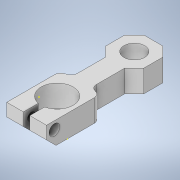
# Autodesk Inventor part: dovetail stabilizer
Saved by Autodesk Inventor 2021 (Build 250183000, 183)
## iProperties
Created: 2020-10-02
Part Number: dovetail stabilizer
Material: Generic
Document SubType Name: Modeling
Designer: User
Density: 1 g/cm^3
Appearance: Default
Author: User
Autodesk Inventor part; units mm, degrees
ref_plane "YZ Plane" through (0, 0, 0) normal (1, 0, 0) x (0, 1, 0)
ref_plane "XZ Plane" through (0, 0, 0) normal (0, 1, 0) x (-1, 0, 0)
ref_plane "XY Plane" through (0, 0, 0) normal (0, 0, 1) x (1, 0, 0)
sketch "Sketch1" plane through (0, 0, 0) normal (0, 1, 0) x (-1, 0, 0)
  line L0 (3.6632, 6.4956) -> (-8.8368, 6.4956)
  line L1 (-8.8368, 6.4956) -> (-8.8368, -10.5044)
  line L2 (-8.8368, -10.5044) -> (3.6632, -10.5044)
  line L3 (3.6632, -10.5044) -> (3.6632, 6.4956)
  line L4 (0.9132, -10.5044) -> (-6.0868, -10.5044)
  point P0 (0, 0)
  dimension "d0" = 17
  dimension "d1" = 12.5
  constraints: 10 end point, 2 horizontal, 2 parallel, 1 perpendicular, 1 point on line
  measures "d0" distance of L2.end L0.start
  measures "d1" distance of L0.start L0.end
extrude "Extrusion1" add sketch "Sketch1" along normal blind 7
chamfer "Chamfer1" distance 3 angle 45 1 edges at (2.5868, 0, 6.4956)
sketch "Sketch2" plane through (0, 7, 0) normal (0, 1, 0) x (1, 0, 0)
  circle A0 centre (2.5868, 3.1044) radius 5.025
  line L0 (8.8368, -6.4956) -> (8.8368, 10.5044) projected
  line L1 (-3.6632, -6.4956) -> (8.8368, -6.4956) projected
  point P0 (0, 0)
  dimension "d7" = 10.05
  dimension "d8" = 6.25
  dimension "d9" = 9.6
  constraints: 1 centre point
  measures "d7" diameter of A0
  measures "d8" distance from line of L0 A0.centre
  measures "d9" distance from line of L1 A0.centre
extrude "Extrusion2" cut sketch "Sketch2" against normal up to next
sketch "Sketch3" plane through (0, 7, 0) normal (0, 1, 0) x (1, 0, 0)
  line L0 (-3.6632, -6.4956) -> (8.8368, -6.4956) projected
  line L1 (1.5868, -6.4956) -> (3.5868, -6.4956)
  line L2 (3.5868, -6.4956) -> (3.5868, 0)
  line L3 (3.5868, 0) -> (1.5868, 0)
  line L4 (1.5868, 0) -> (1.5868, -6.4956)
  line L5 (8.8368, -6.4956) -> (8.8368, 10.5044) projected
  line L6 (-3.6632, 10.5044) -> (-3.6632, -6.4956) projected
  point P0 (0, 0)
  dimension "d16" = 2
  dimension "d17" = 12.5
  dimension "d18" = 5.25
  constraints: 8 end point, 2 parallel, 1 horizontal, 1 perpendicular, 1 point on line
  measures "d16" distance between parallel lines of L2 L4
  measures "d17" distance of L0.start L0.end
  measures "d18" distance between parallel lines of L5 L2
extrude "Extrusion3" cut sketch "Sketch3" against normal through all
sketch "Sketch4" plane through (8.8368, 0, -10.5044) normal (1, 0, 0) x (0, 0, -1)
  line L0 (-17, 3) -> (-17, 7) projected
  line L1 (-17, 7) -> (0, 7) projected
  point P0 (-10.5044, 0)
  point P1 (-14.5, 4.5)
  dimension "d26" = 2.5
  dimension "d27" = 2.5
  measures "d26" distance from line of L0 point (-14.5, 4.5)
  measures "d27" distance from line of L1 point (-14.5, 4.5)
hole "Hole1" at (8.8368, 4.5, 3.9956) direction (-1, 0, 0) diameter 3.4 depth 5.25 clearance for "Flat Head Machine Screw" size "M3" standard "Ansi Metric M Profile"
sketch "Sketch5" plane through (1.5868, 7, 6.4956) normal (1, 0, 0) x (0, 0, -1)
  line L0 (0, 0) -> (17, 0) projected
  line L1 (0, -4) -> (0, 0) projected
  point P0 (6.4956, -7)
  point P1 (2.5, -2.5)
  dimension "d35" = 2.5
  dimension "d36" = 2.5
  measures "d35" distance from line of L0 point (2.5, -2.5)
  measures "d36" distance from line of L1 point (2.5, -2.5)
hole "Hole2" at (1.5868, 4.5, 3.9956) direction (-1, 0, 0) diameter 2.459 depth 5.25 thread size "M3x0.5" class "6H" standard "ANSI Metric M Profile"
sketch "Sketch6" plane through (8.8368, 0, -10.5044) normal (0, 0, -1) x (-1, 0, 0)
  line L0 (5.25, 7) -> (0, 7) projected
  line L1 (3.25, 7) -> (9.25, 7)
  line L2 (9.25, 7) -> (9.25, 0)
  line L3 (9.25, 0) -> (3.25, 0)
  line L4 (3.25, 0) -> (3.25, 7)
  line L5 (0, 0) -> (0, 7) projected
  point P0 (8.8368, 0)
  dimension "d40" = 6
  dimension "d41" = 7
  dimension "d42" = 3.25
  constraints: 8 end point, 2 parallel, 1 horizontal, 1 perpendicular, 1 point on line
  measures "d40" distance of L1.start L1.end
  measures "d41" distance of L3.end L1.start
  measures "d42" distance between parallel lines of L5 L4
extrude "Extrusion4" add sketch "Sketch6" along normal blind 10.85
fillet "Fillet1" radius 2 1 edges at (8.8368, 3.5, -10.5044)
fillet "Fillet2" radius 2 1 edges at (5.5868, 3.5, -10.5044)
fillet "Fillet3" radius 2 2 edges at (-3.6632, 3.5, -10.5044) (-0.4132, 3.5, -10.5044)
sketch "Sketch7" plane through (0, 7, 0) normal (0, 1, 0) x (1, 0, 0)
  point P0 (0, 0)
sketch "Sketch8" plane through (8.8368, 0, -21.3544) normal (0, 0, -1) x (-1, 0, 0)
  point P0 (8.8368, 0)
sketch "Sketch9" plane through (0, 7, 0) normal (0, 1, 0) x (1, 0, 0)
  line L0 (5.5868, 21.3544) -> (-0.4132, 21.3544) projected
  line L1 (5.5868, 21.3544) -> (8.5868, 24.3544)
  line L2 (8.5868, 24.3544) -> (8.5868, 30.3544)
  line L3 (-3.4132, 30.3544) -> (-3.4132, 24.3544)
  line L4 (-3.4132, 24.3544) -> (-0.4132, 21.3544)
  line L5 (8.5868, 30.3544) -> (5.5868, 33.3544)
  line L6 (5.5868, 33.3544) -> (-0.4132, 33.3544)
  line L7 (-0.4132, 33.3544) -> (-3.4132, 30.3544)
  line L8 (5.5868, 12.4335) -> (5.5868, 21.3544) projected
  line L9 (-0.4132, 12.4335) -> (-0.4132, 21.3544) projected
  point P0 (0, 0)
  dimension "d110" = 6
  dimension "d111" = 6
  dimension "d112" = 6
  dimension "d113" = 6
  dimension "d114" = 45
  dimension "d115" = 135
  dimension "d116" = 45
  dimension "d117" = 45
  dimension "d118" = 45
  dimension "d119" = 3
  dimension "d120" = 3
  constraints: 14 end point, 1 horizontal, 1 perpendicular
  measures "d110" distance of L0.start L0.end
  measures "d111" distance of L5.end L6.end
  measures "d112" distance of L1.end L2.end
  measures "d113" distance of L3.start L3.end
  measures "d114" angle of L4 L0
  measures "d115" angle of L1 L0
  measures "d116" angle of L7 L3
  measures "d117" angle of L6 L7
  measures "d118" angle of L5 L6
  measures "d119" horizontal distance of L0.start L1.end
  measures "d120" horizontal distance of L3.end L0.end
extrude "Extrusion5" add sketch "Sketch9" against normal blind 7
sketch "Sketch10" plane through (0, 7, 0) normal (0, 1, 0) x (1, 0, 0)
  circle A0 centre (2.5868, 27.3544) radius 3.25
  line L0 (5.5868, 33.3544) -> (-0.4132, 33.3544) projected
  line L1 (8.5868, 24.3544) -> (8.5868, 30.3544) projected
  line L2 (-3.4132, 30.3544) -> (-3.4132, 24.3544) projected
  point P0 (0, 0)
  dimension "d76" = 6.5
  dimension "d77" = 6
  dimension "d78" = 6
  dimension "d121" = 12
  constraints: 1 centre point
  measures "d76" diameter of A0
  measures "d77" distance from line of L0 A0.centre
  measures "d78" distance from line of L1 A0.centre
  measures "d121" distance between parallel lines of L1 L2
extrude "Extrusion6" cut sketch "Sketch10" against normal up to next
sketch "Sketch11" plane through (8.8368, 3, 6.4956) normal (1, 0, 0) x (0, 0, -1)
  point P0 (6.4956, -3)
sketch "Sketch12" plane through (5.8368, 0, -21.6044) normal (0.7071, 0, 0.7071) x (0.7071, 0, -0.7071)
  line L0 (-0.3536, 7) -> (3.8891, 7) projected
  line L1 (3.8891, 7) -> (3.8891, 0) projected
  point P0 (-19.4039, 0)
  dimension "d122" = 7
  dimension "d123" = 4.2426
  measures "d122" distance of L0.end L1.end
  measures "d123" distance of L0.start L0.end
hole "Hole3" [suppressed]
sketch "Sketch13" plane through (8.5868, 0, -30.3544) normal (0.7071, 0, -0.7071) x (-0.7071, 0, -0.7071)
  line L0 (4.2426, 7) -> (4.2426, 0) projected
  line L1 (4.2426, 0) -> (0, 0) projected
  point P0 (-15.392, 0)
hole "Hole4" [suppressed]
equation "\"d18\" = 0.5 * d17 - 0.5 * d16"
equation "\"d111\" = d110"
equation "\"d112\" = d110"
equation "\"d113\" = d110"
equation "\"d116\" = d114"
equation "\"d117\" = d116"
equation "\"d118\" = d117"
equation "\"d120\" = d119"
equation "\"d77\" = d78"
equation "\"d78\" = 0.5 * d121"
body "Solid1"
